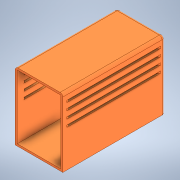
# Autodesk Inventor part: Enclosure
Saved by Autodesk Inventor 2022 (Build 260153000, 153)
## iProperties
Created: 2021-12-24
Part Number: Enclosure
Material: PLA Plastic
Document SubType Name: Modeling
Designer: chad
Density: 0.25 g/cm^3
Appearance: Generic
Author: chad
Autodesk Inventor part; units mm, degrees
ref_plane "YZ Plane" through (0, 0, 0) normal (1, 0, 0) x (0, 1, 0)
ref_plane "XZ Plane" through (0, 0, 0) normal (0, 1, 0) x (-1, 0, 0)
ref_plane "XY Plane" through (0, 0, 0) normal (0, 0, 1) x (1, 0, 0)
sketch "Sketch8" plane through (0, 0, 0) normal (0, 0, 1) x (1, 0, 0)
  line L0 (-17.5, -25) -> (17.5, -25)
  line L1 (17.5, -25) -> (17.5, 25)
  line L2 (17.5, 25) -> (-17.5, 25)
  line L3 (-17.5, 25) -> (-17.5, -25)
  line L4 (-17.5, -25) -> (17.5, 25) construction
  line L5 (17.5, -25) -> (-17.5, 25) construction
  point P0 (0, 0)
  dimension "d14" = 35
  dimension "d15" = 50
  constraints: 12 end point, 2 midpoint, 2 parallel, 1 horizontal, 1 perpendicular
  measures "d14" distance of L2.end L1.end
  measures "d15" distance of L1.end L0.end
extrude "Extrusion3" add sketch "Sketch8" along normal blind 75
shell "Shell2" thickness 1.5 removed faces 1 at (5.8333, -8.3333, 75)
sketch "Sketch9" plane through (0, 0, 0) normal (0, 0, -1) x (-1, 0, 0)
  line L0 (-12.9046, 18.4244) -> (12.8954, 18.4244)
  line L1 (12.8954, 18.4244) -> (12.8954, 4.0244)
  line L2 (12.8954, 4.0244) -> (-12.9046, 4.0244)
  line L3 (-12.9046, 4.0244) -> (-12.9046, 18.4244)
  line L4 (-12.9046, 18.4244) -> (12.8954, 4.0244) construction
  line L5 (12.8954, 18.4244) -> (-12.9046, 4.0244) construction
  point P0 (0, 0)
  point P1 (-0.0046, 11.2244)
  dimension "d19" = 25.8
  dimension "d20" = 14.4
  constraints: 12 end point, 2 midpoint, 2 parallel, 1 horizontal, 1 perpendicular
  measures "d19" distance of L1.end L2.end
  measures "d20" distance of L0.end L1.end
extrude "Extrusion4" cut sketch "Sketch9" against normal blind 8.2625
sketch "Sketch11" plane through (-17.5, -25, 0) normal (-1, 0, 0) x (0, 0, 1)
  line L0 (4.9978, 32.3966) -> (69.9978, 32.3966)
  line L1 (69.9978, 32.3966) -> (69.9978, 33.8966)
  line L2 (69.9978, 33.8966) -> (4.9978, 33.8966)
  line L3 (4.9978, 33.8966) -> (4.9978, 32.3966)
  line L4 (4.9978, 32.3966) -> (69.9978, 33.8966) construction
  line L5 (69.9978, 32.3966) -> (4.9978, 33.8966) construction
  line L6 (5.016, 27.1605) -> (70.016, 27.1605)
  line L7 (70.016, 27.1605) -> (70.016, 28.6605)
  line L8 (5.016, 28.6605) -> (5.016, 27.1605)
  line L9 (5.016, 27.1605) -> (70.016, 28.6605) construction
  line L10 (70.016, 27.1605) -> (5.016, 28.6605) construction
  line L11 (70.016, 28.6605) -> (5.016, 28.6605)
  line L12 (5.0169, 42.9818) -> (70.0169, 42.9818)
  line L13 (70.0169, 42.9818) -> (70.0169, 44.4818)
  line L14 (70.0169, 44.4818) -> (5.0169, 44.4818)
  line L15 (5.0169, 44.4818) -> (5.0169, 42.9818)
  line L16 (5.0169, 42.9818) -> (70.0169, 44.4818) construction
  line L17 (70.0169, 42.9818) -> (5.0169, 44.4818) construction
  line L18 (5.0176, 37.6751) -> (70.0176, 37.6751)
  line L19 (70.0176, 37.6751) -> (70.0176, 39.1751)
  line L20 (5.0176, 39.1751) -> (5.0176, 37.6751)
  line L21 (5.0176, 37.6751) -> (70.0176, 39.1751) construction
  line L22 (70.0176, 37.6751) -> (5.0176, 39.1751) construction
  line L23 (70.0176, 39.1751) -> (5.0176, 39.1751)
  point P0 (0, 25)
  point P1 (37.4978, 33.1466)
  point P2 (37.516, 27.9105)
  point P3 (37.5169, 43.7318)
  point P4 (37.5176, 38.4251)
  dimension "d31" = 65
  dimension "d32" = 1.5
  dimension "d33" = 65
  dimension "d34" = 1.5
  dimension "d35" = 65
  dimension "d36" = 1.5
  dimension "d37" = 65
  dimension "d38" = 1.5
  constraints: 48 end point, 8 midpoint, 8 parallel, 4 horizontal, 4 perpendicular
  measures "d31" distance of L2.end L1.end
  measures "d32" distance of L1.end L0.end
  measures "d33" distance of L11.end L11.start
  measures "d34" distance of L11.start L7.start
  measures "d35" distance of L15.start L14.start
  measures "d36" distance of L14.start L12.end
  measures "d37" distance of L20.start L19.end
  measures "d38" distance of L19.end L18.end
extrude "Extrusion5" cut sketch "Sketch11" against normal blind 1.9125
sketch "Sketch12" plane through (-16, 23.5, 1.5) normal (0, 0, 1) x (1, 0, 0)
  circle A0 centre (16.0592, -33.8393) radius 2.5
  circle A1 centre (16.0592, -33.8393) radius 3.25
  point P0 (16, -23.5)
  dimension "d43" = 5
  dimension "d44" = 6.5
  constraints: 2 centre point, 1 coincident
  measures "d43" diameter of A0
  measures "d44" diameter of A1
extrude "Extrusion7" add sketch "Sketch12" along normal blind 8
sketch "Sketch13" plane through (0.0592, -10.3393, 1.5) normal (0, 0, 1) x (1, 0, 0)
  point P0 (-0.0592, 10.3393)
sketch "Sketch15" plane through (-17.5, -25, 0) normal (0, -1, 0) x (1, 0, 0)
  point P0 (17.5, 0)
sketch "Sketch16" plane through (-16, 23.5, 1.5) normal (0, 0, 1) x (1, 0, 0)
  circle A0 centre (16.0166, -33.7859) radius 2.5072
  point P0 (16, -23.5)
  constraints: 1 centre point
extrude "Extrusion9" cut sketch "Sketch16" against normal blind 1
fillet "Fillet5" radius 2 1 edges at (0, 25, 0)
fillet "Fillet6" radius 2 6 edges at (-17.5, 24.4142, 0.5858) (-17.5, 25, 38.5) (-17.5, -1, 0) (17.5, 24.4142, 0.5858) (17.5, 25, 38.5) (17.5, -1, 0)
fillet "Fillet7" radius 2 8 edges at (-17.5, 18.7318, 5.0169) (-17.5, 13.4251, 5.0176) (-17.5, 8.1466, 4.9978) (-17.5, 2.9105, 5.016) (-17.5, 2.9105, 70.016) (-17.5, 8.1466, 69.9978) (-17.5, 13.4251, 70.0176) (-17.5, 18.7318, 70.0169)
sketch "Sketch17" plane through (17.5, -25, 75) normal (1, 0, 0) x (0, 0, -1)
  line L0 (5.0176, 37.6751) -> (70.0176, 37.6751)
  line L1 (5.0176, 39.1751) -> (5.0176, 37.6751)
  line L2 (70.0176, 37.6751) -> (70.0176, 39.1751)
  line L3 (5.0176, 37.6751) -> (70.0176, 39.1751) construction
  line L4 (70.0176, 37.6751) -> (5.0176, 39.1751) construction
  line L5 (70.0176, 39.1751) -> (5.0176, 39.1751)
  line L6 (5.0169, 42.9818) -> (70.0169, 42.9818)
  line L7 (5.0169, 44.4818) -> (5.0169, 42.9818)
  line L8 (70.0169, 44.4818) -> (5.0169, 44.4818)
  line L9 (70.0169, 42.9818) -> (5.0169, 44.4818) construction
  line L10 (70.0169, 42.9818) -> (70.0169, 44.4818)
  line L11 (5.0169, 42.9818) -> (70.0169, 44.4818) construction
  line L12 (4.9978, 32.3966) -> (69.9978, 32.3966)
  line L13 (69.9978, 32.3966) -> (69.9978, 33.8966)
  line L14 (69.9978, 33.8966) -> (4.9978, 33.8966)
  line L15 (4.9978, 33.8966) -> (4.9978, 32.3966)
  line L16 (4.9978, 32.3966) -> (69.9978, 33.8966) construction
  line L17 (70.016, 28.6605) -> (5.016, 28.6605)
  line L18 (70.016, 27.1605) -> (70.016, 28.6605)
  line L19 (70.016, 27.1605) -> (5.016, 28.6605) construction
  line L20 (5.016, 27.1605) -> (70.016, 27.1605)
  line L21 (5.016, 27.1605) -> (70.016, 28.6605) construction
  line L22 (5.016, 28.6605) -> (5.016, 27.1605)
  line L23 (69.9978, 32.3966) -> (4.9978, 33.8966) construction
  point P0 (75, 25)
  point P1 (0, 25)
  point P2 (37.5176, 38.4251)
  point P3 (37.5169, 43.7318)
  point P4 (37.4978, 33.1466)
  point P5 (37.516, 27.9105)
  dimension "d57" = 65
  dimension "d58" = 1.5
  dimension "d59" = 65
  dimension "d60" = 1.5
  dimension "d61" = 65
  dimension "d62" = 1.5
  dimension "d63" = 65
  dimension "d64" = 1.5
  constraints: 48 end point, 8 midpoint, 8 parallel, 4 horizontal, 4 perpendicular
  measures "d57" distance of L14.end L13.end
  measures "d58" distance of L13.end L12.end
  measures "d59" distance of L17.end L17.start
  measures "d60" distance of L17.start L18.start
  measures "d61" distance of L7.start L8.start
  measures "d62" distance of L8.start L6.end
  measures "d63" distance of L1.start L2.end
  measures "d64" distance of L2.end L0.end
extrude "Extrusion10" cut sketch "Sketch17" against normal blind 5
fillet "Fillet9" radius 2 8 edges at (17.5, 18.7318, 69.9831) (17.5, 13.4251, 69.9824) (17.5, 8.1466, 70.0022) (17.5, 2.9105, 69.984) (17.5, 18.7318, 4.9831) (17.5, 13.4251, 4.9824) (17.5, 8.1466, 5.0022) (17.5, 2.9105, 4.984)
sketch "Sketch18" plane through (-16, 23.5, 1.5) normal (0, 0, 1) x (1, 0, 0)
  line L0 (10, -0.9214) -> (22, -0.9214)
  line L1 (22, -0.9214) -> (22, -3.9214)
  line L2 (22, -3.9214) -> (10, -3.9214)
  line L3 (10, -3.9214) -> (10, -0.9214)
  line L4 (10, -0.9214) -> (22, -3.9214) construction
  line L5 (22, -0.9214) -> (10, -3.9214) construction
  point P0 (16, -23.5)
  point P1 (16, -2.4214)
  dimension "d68" = 12
  dimension "d69" = 3
  constraints: 12 end point, 2 midpoint, 2 parallel, 1 horizontal, 1 perpendicular
  measures "d68" distance of L1.end L2.end
  measures "d69" distance of L0.end L1.end
extrude "Extrusion11" cut sketch "Sketch18" against normal blind 1
fillet "Fillet10" radius 1 4 edges at (12.9046, 11.2244, 0) (-12.8954, 11.2244, 0) (0.0046, 18.4244, 0) (0.0046, 4.0244, 0)
body "Solid2"
